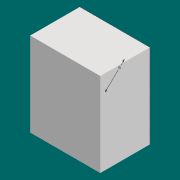
# Autodesk Inventor part: Poti
Saved by Autodesk Inventor 2020.1 (Build 241239000, 239)
## iProperties
Created: 2020-01-27
Part Number: Poti
Material: Generic
Document SubType Name: Modeling
Designer: Pluscrafter
Density: 1 g/cm^3
Appearance: Galvanized
Author: Pluscrafter
Autodesk Inventor part; units mm, degrees
ref_plane "YZ Plane" through (0, 0, 0) normal (1, 0, 0) x (0, 1, 0)
ref_plane "XZ Plane" through (0, 0, 0) normal (0, 1, 0) x (-1, 0, 0)
ref_plane "XY Plane" through (0, 0, 0) normal (0, 0, 1) x (1, 0, 0)
sketch "Sketch1" plane through (0, 0, 0) normal (0, 0, 1) x (1, 0, 0)
  line L0 (0, 0) -> (-9.9, 0)
  line L1 (-9.9, 0) -> (-9.9, 11.87)
  line L2 (-9.9, 11.87) -> (0, 11.87)
  line L3 (0, 11.87) -> (0, 0)
  dimension "d0" = 9.9
  dimension "d1" = 11.87
  constraints: 8 end point, 2 parallel, 1 horizontal, 1 perpendicular
  measures "d0" distance between parallel lines of L3 L1
  measures "d1" distance between parallel lines of L2 L0
extrude "Extrusion1" add sketch "Sketch1" along normal blind 7
sketch "Sketch2" plane through (0, 0, 0) normal (0, 0, -1) x (-1, 0, 0)
  line L0 (9.9, 11.87) -> (9.9, 0) construction
  line L1 (0, 11.87) -> (9.9, 11.87) construction
  line L2 (0, 0) -> (0, 11.87) construction
  line L3 (9.9, 0) -> (0, 0) construction
  line L4 (0, 11.87) -> (9.9, 11.87) construction
  line L5 (4.95, 11.87) -> (4.95, 0) construction
  line L6 (9.9, 11.87) -> (9.9, 0) construction
  line L7 (9.9, 5.935) -> (0, 5.935) construction
  line L8 (0, 0) -> (0, 11.87) construction
  circle A0 centre (4.95, 5.935) radius 3
  dimension "d4" = 6
  constraints: 5 midpoint, 4 end point, 1 centre point
  measures "d4" diameter of A0
extrude "Extrusion2" add sketch "Sketch2" along normal blind 18
body "Solid1"
